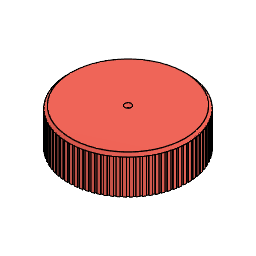
bottlecap tutorial (Autodesk Fusion 360 design; units mm, degrees)
part number: 2025-09-17-15-02-52-867
Autodesk Fusion 360 part; units mm, degrees
sketch "Sketch1" plane through (0, 0, 0) normal (0, 0, 1) x (1, 0, 0)
  circle A0 centre (0, 0) radius 16
  dimension "d11" = 32
  constraint coincident A0.centre origin
  measures "d11" diameter of A0
sketch "Sketch2" plane through (0, 0, 0) normal (0, 0, 1) x (1, 0, 0)
  circle A0 centre (0, 0) radius 16
  dimension "d16" = 32
  constraint coincident A0.centre origin
  measures "d16" diameter of A0
extrude "Extrude2" add sketch "Sketch2" along normal blind 10
chamfer "Chamfer2" distance 0.7 angle 45 1 edges at (-14.9172, -5.7858, 10)
shell "Shell2" thickness 2 removed faces 1 at (3.3126, -0.5422, 0)
thread "Thread1" "ISO Metric profile 30.0 M30x1.5 M30x1.5 6H" major diameter 30.208 minor diameter 28.526 pitch 1.5 angle 60 modelled right hand crest width 0.4036 on face at (13.9304, 1.3939, 5.3333) crest through (14.263, 0, 0.375)
sketch "Sketch3" plane through (0, 0, 10) normal (0, 0, 1) x (-1, 0, 0)
  circle A0 centre (0, 0) radius 15.3
  circle A1 centre (0, 0) radius 0.9
  dimension "d23" = 1.8
  constraint coincident A0.centre A1.centre
  measures "d23" diameter of A1
extrude "Extrude3" cut sketch "Sketch3" against normal blind 0.5 contours A1
fillet "Fillet1" radius 0.9 1 faces at (0.2108, -0.6634, 9.5)
sketch "Sketch4" plane through (0, 0, 0) normal (0, 0, 1) x (1, 0, 0)
  line L0 (-16.8, -0.25) -> (-15.8, -0.25)
  line L1 (-15.8, -0.25) -> (-15.8, 0.25)
  line L2 (-15.8, 0.25) -> (-16.8, 0.25)
  line L3 (-16.8, 0.25) -> (-16.8, -0.25)
  point P0 (-15.3, 0)
  dimension "d28" = 15.8
  dimension "d29" = 0.5
  dimension "d30" = 0.25
  dimension "d31" = 1
  constraint horizontal L0
  constraint vertical L1
  constraint horizontal L2
  constraint vertical L3
  measures "d28" distance of origin L1
  measures "d29" distance of L0.start L2.end
  measures "d30" vertical distance of L0.end P0
  measures "d31" distance of L1.end L3
extrude "Extrude4" cut sketch "Sketch4" along normal blind 9.3
pattern_circular "C-Pattern1" count 80 over 360 about axis through (0, 0, 0) along (0, 0, 1) of "Extrude4"
